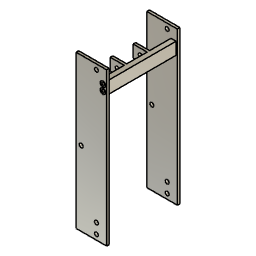
Suspension Plate v10 (Autodesk Fusion 360 design; units mm, degrees)
Autodesk Fusion 360 part; units mm, degrees
sketch "Sketch1" plane through (0, 0, 0) normal (0, 1, 0) x (1, 0, 0)
  line L0 (-12.7, 12.7) -> (63.5, 12.7)
  line L1 (63.5, 12.7) -> (63.5, -368.3)
  line L2 (63.5, -368.3) -> (-12.7, -368.3)
  line L3 (-12.7, -368.3) -> (-12.7, 12.7)
  line L4 (60.325, -340.36) -> (47.625, -340.36)
  line L5 (47.625, -340.36) -> (47.625, -309.88)
  line L6 (47.625, -309.88) -> (60.325, -309.88)
  line L7 (60.325, -309.88) -> (60.325, -340.36)
  line L8 (47.625, -325.12) -> (60.325, -325.12)
  circle A0 centre (38.1, -25.4) radius 4.953
  circle A1 centre (0, -172.9607) radius 4.953
  line L9 (47.625, -325.12) -> (47.625, -340.36) construction
  line L10 (47.625, -325.12) -> (47.625, -309.88) construction
  circle A2 centre (53.975, -332.74) radius 3.175
  circle A3 centre (53.975, -317.5) radius 3.175
  line L11 (53.975, -340.36) -> (53.975, -309.88) construction
  line L12 (47.625, -332.74) -> (57.15, -332.74) construction
  line L13 (47.625, -317.5) -> (57.15, -317.5) construction
  point P0 (47.625, -332.74)
  point P1 (53.975, -340.36)
  point P2 (53.975, -332.74)
  point P3 (47.625, -317.5)
  point P4 (53.975, -309.88)
  point P5 (53.975, -317.5)
  dimension "d11" = 76.2
  dimension "d57" = 9.906
  dimension "d58" = 9.906
  dimension "d59" = 50.8
  dimension "d60" = 38.1
  dimension "d61" = 12.7
  dimension "d62" = 152.4
  dimension "d83" = 381
  dimension "d85" = 30.48
  dimension "d86" = 353.06
  dimension "d87" = 6.35
  dimension "d88" = 6.35
  dimension "d97" = 9.525
  constraint horizontal L0
  constraint vertical L1
  constraint horizontal L2
  constraint vertical L3
  constraint horizontal L4
  constraint vertical L5
  constraint horizontal L6
  constraint vertical L7
  constraint midpoint L5 L8.start
  constraint midpoint L7 L8.end
  constraint midpoint L9 P0
  constraint midpoint L4 P1
  constraint midpoint L10 P3
  constraint midpoint L6 P4
  constraint coincident P2 A2.centre
  constraint coincident P5 A3.centre
  constraint coincident P1 L11.start
  constraint coincident P4 L11.end
  constraint coincident P0 L12.start
  constraint coincident A2 L12.end
  constraint perpendicular L11 L12
  constraint coincident P3 L13.start
  constraint coincident A3 L13.end
  constraint perpendicular L7 L13
  measures "d11" distance of L0.start L0.end
  measures "d57" diameter of A0
  measures "d58" diameter of A1
  measures "d59" distance of L3 A0.centre
  measures "d60" distance of L0 A0.centre
  measures "d61" distance of L3 A1.centre
  measures "d62" distance of A0.centre A1.centre
  measures "d83" distance of L0 L2
  measures "d85" distance of L4 L6
  measures "d86" distance of L0 L4
  measures "d87" diameter of A2
  measures "d88" diameter of A3
  measures "d97" distance of L1 P1
extrude "Extrude1" add sketch "Sketch1" along normal blind 5.08 contours L0 L1 L2 L3 | L4 L5 L7 L8 | L5 L6 L7 L8 | A2 | A3
extrude "Extrude3" add sketch "Sketch1" against normal blind 170.18 contours L4 L5 L7 L8 | L5 L6 L7 L8 | A2 | A3
sketch "Sketch2" plane through (47.625, 0, 0) normal (-1, 0, 0) x (0, -1, 0)
  line L0 (0, 340.36) -> (0, 309.88)
  line L1 (0, 309.88) -> (170.18, 309.88)
  line L2 (170.18, 309.88) -> (170.18, 340.36)
  line L3 (170.18, 340.36) -> (0, 340.36)
  line L4 (85.09, 309.88) -> (85.09, 340.36)
  line L5 (170.18, 325.12) -> (0, 325.12)
  line L6 (59.69, 320.3575) -> (110.49, 320.3575) construction
  line L7 (110.49, 320.3575) -> (110.49, 329.8825) construction
  line L8 (110.49, 329.8825) -> (59.69, 329.8825) construction
  line L9 (59.69, 329.8825) -> (59.69, 320.3575) construction
  line L10 (59.69, 325.12) -> (110.49, 325.12)
  line L11 (85.09, 329.8825) -> (85.09, 320.3575)
  line L12 (110.49, 340.36) -> (115.57, 340.36)
  line L13 (115.57, 340.36) -> (115.57, 309.88)
  line L14 (115.57, 309.88) -> (110.49, 309.88)
  line L15 (110.49, 309.88) -> (110.49, 340.36)
  line L16 (54.61, 340.36) -> (54.61, 309.88)
  line L17 (59.69, 309.88) -> (59.69, 340.36)
  line L18 (59.69, 340.36) -> (54.61, 340.36)
  line L19 (54.61, 309.88) -> (59.69, 309.88)
  dimension "d26" = 9.525
  dimension "d27" = 50.8
  dimension "d28" = 30.48
  dimension "d29" = 85.09
  dimension "d30" = 5.08
  dimension "d31" = 5.08
  dimension "d32" = 30.48
  constraint midpoint L1 L4.start
  constraint midpoint L3 L4.end
  constraint midpoint L2 L5.start
  constraint midpoint L0 L5.end
  constraint horizontal L6
  constraint vertical L7
  constraint horizontal L8
  constraint vertical L9
  constraint midpoint L9 L10.start
  constraint midpoint L7 L10.end
  constraint midpoint L8 L11.start
  constraint midpoint L6 L11.end
  constraint horizontal L12
  constraint vertical L13
  constraint horizontal L14
  constraint vertical L15
  constraint coincident L3 L12.start
  constraint symmetric L4 L12.start L17.end
  constraint symmetric L4 L12.end L16.start
  constraint symmetric L4 L13.end L16.end
  constraint symmetric L4 L14.end L17.start
  measures "d26" distance of L6.start L8.end
  measures "d27" distance of L6.start L6.end
  measures "d29" distance of L2 L11
  measures "d30" distance of L12.start L12.end
  measures "d31" distance of L7 L13
  measures "d32" distance of L12.end L13.end
extrude "Extrude4" add sketch "Sketch2" along normal blind 34.925 contours L3 L5 L16 L17 L18 | L1 L5 L16 L17 L19 | L3 L5 L12 L13 L15 | L1 L5 L13 L14 L15
hole "Hole1" at (30.1625, -59.69, 325.12) direction (0, 1, 0) diameter 9.525 depth 10.16 tip angle 118
hole "Hole2" at (30.1625, -115.57, 325.12) direction (0, 1, 0) diameter 9.525 depth 10.16 tip angle 118
sketch "Sketch3" plane through (0, -170.18, 0) normal (0, -1, 0) x (1, 0, 0)
  line L0 (47.625, 309.88) -> (60.325, 309.88)
  line L1 (60.325, 309.88) -> (60.325, 340.36)
  line L2 (60.325, 340.36) -> (47.625, 340.36)
  line L3 (47.625, 340.36) -> (47.625, 309.88)
  line L4 (63.4581, 368.3) -> (-12.7419, 368.3)
  line L5 (-12.7419, 368.3) -> (-12.7419, -12.7)
  line L6 (-12.7419, -12.7) -> (63.4581, -12.7)
  line L7 (63.4581, -12.7) -> (63.4581, 368.3)
  circle A0 centre (38.0581, 25.4) radius 4.953
  circle A1 centre (-0.0419, 172.9607) radius 4.953
  dimension "d41" = 381
  dimension "d42" = 76.2
  dimension "d45" = 9.906
  dimension "d48" = 9.906
  dimension "d63" = 38.1
  dimension "d64" = 50.8
  dimension "d65" = 12.7
  dimension "d66" = 152.4
  constraint horizontal L4
  constraint vertical L5
  constraint horizontal L6
  constraint vertical L7
  measures "d41" distance of L6.end L4.start
  measures "d42" distance of L4.end L4.start
  measures "d45" diameter of A0
  measures "d48" diameter of A1
  measures "d63" distance of L6 A0.centre
  measures "d64" distance of L5 A0.centre
  measures "d65" distance of L5 A1.centre
  measures "d66" distance of A0.centre A1.centre
extrude "Extrude5" add 1 faces at (17.2477, 5.08, 304.8077) along direction (0, 1, 0) blind 1.27
extrude "Extrude6" add 1 faces at (43.3872, -54.61, 325.0014) along direction (0, 1, 0) blind 1.27
extrude "Extrude7" add 1 faces at (43.3872, -115.57, 325.2386) along direction (0, -1, 0) blind 1.27
extrude "Extrude8" add sketch "Sketch3" along normal blind 6.35 contours L0 L1 L2 L3 | L4 L5 L6 L7
sketch "Sketch4" plane through (0, -176.53, 0) normal (0, -1, 0) x (1, 0, 0)
  circle A0 centre (-0.0419, 172.9607) radius 4.953
  circle A1 centre (38.0581, 25.4) radius 4.953
  line L0 (63.4581, -12.7) -> (63.4581, 368.3)
  line L1 (63.4581, 368.3) -> (-12.7419, 368.3)
  line L2 (-12.7419, 368.3) -> (-12.7419, -12.7)
  line L3 (-12.7419, -12.7) -> (63.4581, -12.7)
  circle A2 centre (38.0581, 355.6) radius 4.826
  circle A3 centre (38.0581, 0) radius 4.826
  dimension "d67" = 9.652
  dimension "d68" = 25.4
  dimension "d69" = 12.7
  dimension "d70" = 9.652
  dimension "d71" = 25.4
  dimension "d72" = 12.7
  measures "d67" diameter of A2
  measures "d68" distance of L0 A2.centre
  measures "d69" distance of L1 A2.centre
  measures "d70" diameter of A3
  measures "d71" distance of L0 A3.centre
  measures "d72" distance of L3 A3.centre
extrude "Extrude9" cut sketch "Sketch4" against normal blind 6.35 contours A2 | A3
sketch "Sketch5" plane through (0, 6.35, 0) normal (0, 1, 0) x (-1, 0, 0)
  circle A0 centre (-38.1, 25.4) radius 4.953
  circle A1 centre (0, 172.9607) radius 4.953
  line L0 (-63.5, 368.3) -> (-63.5, -12.7)
  line L1 (-63.5, -12.7) -> (12.7, -12.7)
  line L2 (12.7, -12.7) -> (12.7, 368.3)
  line L3 (12.7, 368.3) -> (-63.5, 368.3)
  circle A2 centre (-38.1, 355.6) radius 4.826
  circle A3 centre (-38.1, 0) radius 4.826
  dimension "d75" = 9.652
  dimension "d76" = 12.7
  dimension "d77" = 25.4
  dimension "d78" = 9.652
  dimension "d79" = 25.4
  dimension "d80" = 12.7
  measures "d75" diameter of A2
  measures "d76" distance of L3 A2.centre
  measures "d77" distance of L0 A2.centre
  measures "d78" diameter of A3
  measures "d79" distance of L0 A3.centre
  measures "d80" distance of L1 A3.centre
extrude "Extrude10" cut sketch "Sketch5" against normal blind 6.35 contours A2 | A3
extrude "Extrude11" cut sketch "Sketch1" along normal blind 6.35 and the other way blind 177.8 contours A2 | A3
sketch "Sketch6" plane through (0, -176.53, 0) normal (0, -1, 0) x (1, 0, 0)
  circle A0 centre (53.975, 332.74) radius 3.175
  circle A1 centre (53.975, 317.5) radius 3.175
  circle A2 centre (38.0581, 355.6) radius 4.826
  circle A3 centre (38.0581, 0) radius 4.826
  circle A4 centre (-0.0419, 172.9607) radius 4.953
  circle A5 centre (38.0581, 25.4) radius 4.953
  line L0 (63.4581, -12.7) -> (63.4581, 368.3)
  line L1 (63.4581, 368.3) -> (-12.7419, 368.3)
  line L2 (-12.7419, 368.3) -> (-12.7419, -12.7)
  line L3 (-12.7419, -12.7) -> (63.4581, -12.7)
  circle A6 centre (53.975, 332.74) radius 6.7437
  circle A7 centre (53.975, 317.5) radius 6.7437
  dimension "d93" = 13.4874
  dimension "d94" = 13.4874
  constraint concentric A0 A6
  constraint concentric A1 A7
  measures "d93" diameter of A6
  measures "d94" diameter of A7
extrude "Extrude12" cut sketch "Sketch6" against normal blind 1.27 contours A6 | A7
equation "d26 = ( 3 / 8 ) * 1 in"
equation "d65 = ( 1 / 2 ) * 1 in"
equation "d73 = ( -1 / 4 ) * 1 in"
equation "d81 = ( -1 / 4 ) * 1 in"
equation "d87 = ( 1 / 4 ) * 1 in"
equation "d88 = ( 1 / 4 ) * 1 in"
equation "d89 = 1 / 4 * in"
equation "d97 = ( 3 / 8 ) * 1 in"
